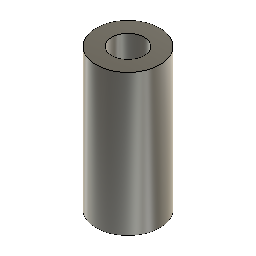
syringe-adapter v5 (Autodesk Fusion 360 design; units mm, degrees)
Autodesk Fusion 360 part; units mm, degrees
sketch "tip bottom" plane through (0, 0, 0) normal (0, 0, 1) x (1, 0, 0)
  circle A0 centre (0, 0) radius 2.5
  dimension "d2" = 5
  constraint coincident A0.centre origin
  measures "d2" diameter of A0
ref_plane "WorkPlane1" through (0, 0, 8.1) normal (0, 0, 1) x (1, 0, 0)
sketch "tip top" plane through (0, 0, 8.1) normal (0, 0, 1) x (1, 0, 0)
  circle A0 centre (0, 0) radius 2.3
  dimension "d5" = 4.6
  constraint coincident A0.centre origin
  measures "d5" diameter of A0
loft "Loft1" add profiles "tip top", "tip bottom" section 1 section 2 makes body 1
sketch "od sketch and bore hole" plane through (0, 0, 0) normal (0, 0, 1) x (1, 0, 0)
  circle A0 centre (0, 0) radius 4.5
  circle A1 centre (0, 0) radius 2.3
  dimension "d6" = 9
  dimension "d9" = 4.6
  constraint coincident A0.centre A1.centre
  measures "d6" diameter of A0
  measures "d9" diameter of A1
extrude "Extrude1" add sketch "od sketch and bore hole" along normal blind 20 separate body contours A0 | A1 makes body 2
combine "Combine1" operation cut target body 2 tool bodies 1 keep tools
extrude "Extrude2" cut sketch "od sketch and bore hole" along normal blind 40 contours A1 bodies 2
hidden bodies 1
equation "d2 = 4.5 mm + tip_id_plus"
equation "d5 = 4.1 mm + tip_id_plus"
equation "d6 = od"
equation "d9 = 4.1 mm + tip_id_plus"
equation "od = 9.0 mm"
equation "tip_id_plus = 0.5 mm"
named bodies: "neg tip", "outer"
